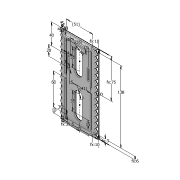
# Autodesk Inventor part: tray
Saved by Autodesk Inventor 2022 (Build 260153000, 153)
## iProperties
Created: 2022-05-19
Part Number: tray
Material: Generic
Document SubType Name: Modeling
Designer: Thomas
Density: 1 g/cm^3
Appearance: Default
Author: Thomas
Autodesk Inventor part; units mm, degrees
ref_plane "YZ Plane" through (0, 0, 0) normal (1, 0, 0) x (0, 1, 0)
ref_plane "XZ Plane" through (0, 0, 0) normal (0, 1, 0) x (-1, 0, 0)
ref_plane "XY Plane" through (0, 0, 0) normal (0, 0, 1) x (1, 0, 0)
sketch "Sketch1" plane through (0, 0, 0) normal (0, 0, 1) x (1, 0, 0)
  line L0 (0, 0) -> (71, 0)
  line L1 (71, 0) -> (71, -150)
  line L2 (71, -150) -> (0, -150)
  line L3 (0, -150) -> (0, 0)
  line L4 (7.6868, 0) -> (92.3291, 0)
  line L5 (9.7325, -150) -> (92.3291, -150)
  line L6 (9.7325, -150) -> (11.7224, -150)
  line L7 (0, 0) -> (5, -5)
  line L8 (0, 0) -> (7.0711, 0) construction
  line L9 (5, -5) -> (0, -10)
  line L10 (0, -10) -> (5, -15)
  line L11 (5, -15) -> (0, -20)
  line L12 (0, -20) -> (5, -25)
  line L13 (5, -25) -> (0, -30)
  line L14 (0, -30) -> (5, -35)
  line L15 (5, -35) -> (0, -40)
  line L16 (0, -40) -> (5, -45)
  line L17 (5, -45) -> (0, -50)
  line L18 (0, -50) -> (5, -55)
  line L19 (5, -55) -> (0, -60)
  line L20 (0, -60) -> (5, -65)
  line L21 (5, -65) -> (0, -70)
  line L22 (0, -70) -> (5, -75)
  line L23 (5, -75) -> (0, -80)
  line L24 (0, -80) -> (5, -85)
  line L25 (5, -85) -> (0, -90)
  line L26 (0, -90) -> (5, -95)
  line L27 (5, -95) -> (0, -100)
  line L28 (0, -100) -> (5, -105)
  line L29 (5, -105) -> (0, -110)
  line L30 (0, -110) -> (5, -115)
  line L31 (5, -115) -> (0, -120)
  line L32 (0, -120) -> (5, -125)
  line L33 (5, -125) -> (0, -130)
  line L34 (0, -130) -> (5, -135)
  line L35 (5, -135) -> (0, -140)
  line L36 (35.5, 0) -> (35.5, -140) construction
  line L37 (71, 0) -> (66, -5)
  line L38 (66, -5) -> (71, -10)
  line L39 (71, -10) -> (66, -15)
  line L40 (66, -15) -> (71, -20)
  line L41 (71, -20) -> (66, -25)
  line L42 (66, -25) -> (71, -30)
  line L43 (71, -30) -> (66, -35)
  line L44 (66, -35) -> (71, -40)
  line L45 (71, -40) -> (66, -45)
  line L46 (66, -45) -> (71, -50)
  line L47 (71, -50) -> (66, -55)
  line L48 (66, -55) -> (71, -60)
  line L49 (71, -60) -> (66, -65)
  line L50 (66, -65) -> (71, -70)
  line L51 (71, -70) -> (66, -75)
  line L52 (66, -75) -> (71, -80)
  line L53 (71, -80) -> (66, -85)
  line L54 (66, -85) -> (71, -90)
  line L55 (71, -90) -> (66, -95)
  line L56 (66, -95) -> (71, -100)
  line L57 (71, -100) -> (66, -105)
  line L58 (66, -105) -> (71, -110)
  line L59 (71, -110) -> (66, -115)
  line L60 (66, -115) -> (71, -120)
  line L61 (71, -120) -> (66, -125)
  line L62 (66, -125) -> (71, -130)
  line L63 (71, -130) -> (66, -135)
  line L64 (66, -135) -> (71, -140)
  line L65 (10, -3) -> (61, -3)
  line L66 (61, -3) -> (61, -6)
  line L67 (61, -6) -> (10, -6)
  line L68 (10, -6) -> (10, -3)
  line L69 (10, -144) -> (61, -144)
  line L70 (61, -144) -> (61, -147)
  line L71 (61, -147) -> (10, -147)
  line L72 (10, -147) -> (10, -144)
  line L73 (0, -140) -> (5, -145)
  line L74 (5, -145) -> (0, -150)
  line L75 (66, -5) -> (71, -10)
  line L76 (71, -140) -> (66, -145)
  line L77 (66, -145) -> (71, -150)
  line L78 (11, -80) -> (11, -140) construction
  line L79 (9.4, -80) -> (9.4, -140)
  line L80 (12.6, -140) -> (12.6, -80)
  arc A0 (12.6, -80) -> (9.4, -80) centre (11, -80) ccw
  arc A1 (9.4, -140) -> (12.6, -140) centre (11, -140) ccw
  line L81 (16.5, -40) -> (16.5, -60) construction
  line L82 (15, -40) -> (15, -60)
  line L83 (18, -60) -> (18, -40)
  arc A2 (18, -40) -> (15, -40) centre (16.5, -40) ccw
  arc A3 (15, -60) -> (18, -60) centre (16.5, -60) ccw
  line L84 (54.5, -40) -> (54.5, -60) construction
  line L85 (56, -40) -> (56, -60)
  line L86 (53, -60) -> (53, -40)
  arc A4 (56, -40) -> (53, -40) centre (54.5, -40) ccw
  arc A5 (53, -60) -> (56, -60) centre (54.5, -60) ccw
  line L87 (60, -80) -> (60, -140) construction
  line L88 (61.6, -80) -> (61.6, -140)
  line L89 (58.4, -140) -> (58.4, -80)
  arc A6 (61.6, -80) -> (58.4, -80) centre (60, -80) ccw
  arc A7 (58.4, -140) -> (61.6, -140) centre (60, -140) ccw
  line L90 (35.5, -129) -> (35.5, -94) construction
  line L91 (43, -129) -> (43, -94)
  line L92 (28, -94) -> (28, -129)
  arc A8 (28, -129) -> (43, -129) centre (35.5, -129) ccw
  arc A9 (43, -94) -> (28, -94) centre (35.5, -94) ccw
  line L93 (35.5, -56) -> (35.5, -21) construction
  line L94 (43, -56) -> (43, -21)
  line L95 (28, -21) -> (28, -56)
  arc A10 (28, -56) -> (43, -56) centre (35.5, -56) ccw
  arc A11 (43, -21) -> (28, -21) centre (35.5, -21) ccw
  line L96 (71, -75) -> (0, -75) construction
  line L97 (11, -70) -> (11, -10) construction
  line L98 (9.4, -70) -> (9.4, -10)
  line L99 (12.6, -10) -> (12.6, -70)
  arc A12 (9.4, -70) -> (12.6, -70) centre (11, -70) ccw
  arc A13 (12.6, -10) -> (9.4, -10) centre (11, -10) ccw
  line L100 (61.6, -70) -> (61.6, -10)
  line L101 (58.4, -10) -> (58.4, -70)
  line L102 (60, -70) -> (60, -10) construction
  arc A14 (61.6, -10) -> (58.4, -10) centre (60, -10) ccw
  arc A15 (58.4, -70) -> (61.6, -70) centre (60, -70) ccw
  point P0 (11, -110)
  point P1 (16.5, -50)
  point P2 (54.5, -50)
  point P3 (60, -110)
  point P4 (35.5, -111.5)
  point P5 (35.5, -38.5)
  point P6 (11, -40)
  point P7 (60, -40)
  dimension "d0" = 71
  dimension "d1" = 150
  dimension "d2" = 45
  dimension "d3" = 5
  dimension "d6" = 10
  dimension "d11" = 35.5
  dimension "d12" = 10
  dimension "d13" = 10
  dimension "d14" = 3
  dimension "d15" = 10
  dimension "d16" = 3
  dimension "d17" = 138
  dimension "d19" = 6
  dimension "d20" = 3.2
  dimension "d21" = 11
  dimension "d22" = 10
  dimension "d24" = 51
  dimension "d25" = 3
  dimension "d26" = 4
  dimension "d27" = 40
  dimension "d28" = 20
  dimension "d29" = 35
  dimension "d30" = 41
  dimension "d36" = 35
  dimension "d37" = 15
  dimension "d38" = 15
  dimension "d39" = 35
  dimension "d40" = 15
  dimension "d41" = 15
  dimension "d44" = 60
  dimension "d45" = 75
  constraints: 222 end point, 73 symmetric about line, 32 point on circle, 16 centre point, 16 tangent, 10 parallel, 9 point on line, 7 horizontal, 6 midpoint, 6 perpendicular, 3 vertical, 1 equal length, 78 other
  measures "d0" distance of L1.end L2.end
  measures "d1" distance of L0.end L1.end
  measures "d2" angle of L7 L8
  measures "d3" horizontal distance of L0.start L7.end
  measures "d6" distance of L0.start L10.start
  measures "d11" distance between parallel lines of L3 L36
  measures "d12" distance between parallel lines of L3 L68
  measures "d13" distance between parallel lines of L1 L66
  measures "d14" distance between parallel lines of L67 L65
  measures "d15" distance between parallel lines of L1 L70
  measures "d16" distance between parallel lines of L69 L71
  measures "d17" distance between parallel lines of L67 L69
  measures "d19" distance between parallel lines of L5 L69
  measures "d20" diameter of A1
  measures "d21" distance between parallel lines of L3 L78
  measures "d22" distance from line of L2 L78.end
  measures "d24" distance of L65.start L65.end
  measures "d25" diameter of A3
  measures "d26" distance between parallel lines of L82 L78
  measures "d27" distance from line of L0 L81.start
  measures "d28" distance of L81.start L81.end
  measures "d29" distance between parallel lines of L83 L86
  measures "d30" distance between parallel lines of L85 L82
  measures "d36" distance of L90.start L90.end
  measures "d37" diameter of A9
  measures "d38" distance from line of L69 L90.start
  measures "d39" distance of L93.start L93.end
  measures "d40" diameter of A11
  measures "d41" distance from line of L93.end L67
  measures "d44" distance of L78.start L78.end
  measures "d45" distance between parallel lines of L96 L0
extrude "Extrusion1" add sketch "Sketch1" along normal blind 2.5 contours L0 L37 L38 L39 L40 L41 L42 L43 L44 L45 L46 L47 L48 L49 L50 L51 L52 L53 L54 L55 L56 L57 L58 L59 L60 L61 L62 L63 L64 L76 L77 L2 L74 L73 L35 L34 L33 L32 L31 L30 L29 L28 L27 L26 L25 L24 L23 L22 L21 L20 L19 L18 L17 L16 L15 L14 L13 L12 L11 L10 L9 L7 | L65 L66 L67 L68 | L69 L70 L71 L72 | A8 L92 A9 L91 | A10 L95 A11 L94 | L98 A13 L99 A12 | A15 L101 A14 L100
extrude "Extrusion2" add sketch "Sketch1" along normal blind 8 contours L65 L66 L67 L68 | L69 L70 L71 L72
fillet "Fillet1" radius 3 2 edges at (35.5, -147, 2.5) (35.5, -3, 2.5)
extrude "Extrusion3" cut sketch "Sketch1" along normal through all contours A8 L92 A9 L91 | A10 L95 A11 L94
extrude "Extrusion4" cut sketch "Sketch1" along normal through all contours L98 A13 L99 A12 | A15 L101 A14 L100
equation "\"d11\" = 0.5 * d0"
equation "\"d13\" = d12"
equation "\"d15\" = d12"
equation "\"d16\" = d14"
equation "\"d19\" = -0.5 * d17 + 0.5 * d1"
equation "\"d45\" = 0.5 * d1"
body "Solid1"
